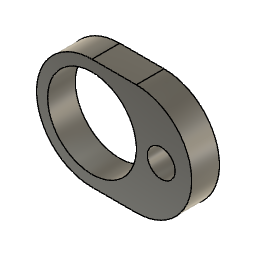
Brazo 1 Nueva Versión v3 (Autodesk Fusion 360 design; units mm, degrees)
Autodesk Fusion 360 part; units mm, degrees
note: some values were not read from the file. Set by a fixed rule: which sketch regions a step uses.
sketch "Boceto1" plane through (0, 0, 0) normal (0, 1, 0) x (1, 0, 0)
  circle A0 centre (0, 0) radius 10
  circle A1 centre (0, 0) radius 2.5
  circle A2 centre (0, 0) radius 8
  line L0 (0, 0) -> (12.5, 0)
  circle A3 centre (12.5, 0) radius 2.5
  line L1 (12.5, -10) -> (0, -10)
  line L2 (0, 10) -> (12.5, 10)
  circle A4 centre (8, 0) radius 10
  dimension "d1" = 5
  dimension "d5" = 16
  dimension "d7" = 12.5
  constraint coincident A0.centre A1.centre
  constraint concentric A1 A2
  constraint horizontal L0
  constraint coincident L0.end A3.centre
  constraint tangent A0 A3
  constraint coincident A0 L1.end
  constraint tangent A0 L1
  constraint horizontal L1
  constraint coincident A0 L2.start
  constraint coincident L0 A4.centre
  constraint tangent L1 A4
  measures "d1" diameter of A1
  measures "d5" diameter of A2
  measures "d7" distance of A0.centre L0.end
extrude "Extruir1" add sketch "Boceto1" along normal blind 5 contours A0 A2 A4 | A0 L2 A4 | A0 L1 A4 | A0 A4 | A0 A2 L0 A4 | A0 A2 L0 A4
ref_plane "PlanoDeObra1" through (-10, 2.3987, 0) normal (-1, 0, 0) x (0, 0, -1)
ref_plane "PlanoDeObra2" through (18, 2.3524, 0) normal (1, 0, 0) x (0, 0, 1)
sketch "Boceto2" plane through (0, 0, 0) normal (0, -1, 0) x (1, 0, 0)
  circle A0 centre (0, 0) radius 8
  circle A1 centre (12.5, 0) radius 2.5
  arc A2 (0, 10) -> (0, -10) centre (0, 0) ccw
  line L0 (0, -10) -> (8, -10)
  arc A3 (8, -10) -> (8, 10) centre (8, 0) ccw
  line L1 (8, 10) -> (0, 10)
  circle A4 centre (12.5, 0) radius 2.5
  dimension "d11" = 5
  constraint concentric A1 A4
  measures "d11" diameter of A4
